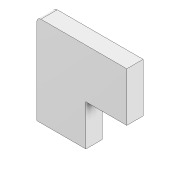
# Autodesk Inventor part: Acolpe L para Soporte LED
Saved by Autodesk Inventor 2020 (Build 240168000, 168)
## iProperties
Created: 2020-08-13
Part Number: Acolpe L para Soporte LED
Material: Acetal Resin, White
Document SubType Name: Modeling
Designer: Dante
Density: 1.425 g/cm^3
Appearance: Smooth - White
Author: Dante
Autodesk Inventor part; units mm, degrees
ref_plane "YZ Plane" through (0, 0, 0) normal (1, 0, 0) x (0, 1, 0)
ref_plane "XZ Plane" through (0, 0, 0) normal (0, 1, 0) x (-1, 0, 0)
ref_plane "XY Plane" through (0, 0, 0) normal (0, 0, 1) x (1, 0, 0)
sketch "Sketch1" plane through (0, 0, 0) normal (0, 0, 1) x (1, 0, 0)
  line L0 (-13.7567, 1.1084) -> (10.2433, 1.1084)
  line L1 (10.2433, 1.1084) -> (10.2433, 21.1084)
  line L2 (10.2433, 21.1084) -> (30.2433, 21.1084)
  line L3 (30.2433, 21.1084) -> (30.2433, 45.1084)
  line L4 (30.2433, 45.1084) -> (-13.7567, 45.1084)
  line L5 (-13.7567, 45.1084) -> (-13.7567, 1.1084)
  dimension "d1" = 24
  dimension "d2" = 20
  dimension "d3" = 20
  dimension "d4" = 24
  constraints: 12 end point, 3 horizontal, 2 perpendicular, 1 vertical
  measures "d1" distance of L0.start L0.end
  measures "d2" distance of L0.end L1.end
  measures "d3" distance of L1.end L2.end
  measures "d4" distance of L2.end L3.end
extrude "Extrusion1" add sketch "Sketch1" along normal blind 8
fillet "Fillet1" radius 2 1 edges at (-13.7567, 45.1084, 4)
equation "\"d4\" = d1"
body "Solid1"
